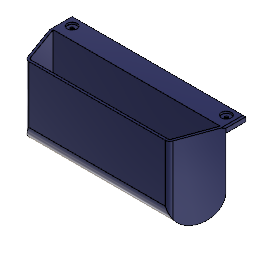
1-Drip tray V3 v4 (Autodesk Fusion 360 design; units mm, degrees)
Autodesk Fusion 360 part; units mm, degrees
mesh "Mesh5" [no effect]
sketch "Sketch3" plane through (0, 0, 10) normal (0, 0, 1) x (-1, 0, 0)
  circle A0 centre (-105, -250) radius 2.75
  circle A1 centre (105, 250) radius 2.75
  circle A2 centre (-105, 250) radius 2.75
  circle A3 centre (105, -250) radius 2.75
  line L0 (-95.6031, -253.4202) -> (-74.3399, -195)
  line L1 (-74.3399, -195) -> (74.3399, -195)
  line L2 (74.3399, -195) -> (95.6031, -253.4202)
  arc A4 (95.6031, -253.4202) -> (115, -250) centre (105, -250) ccw
  line L3 (115, -250) -> (115, 250)
  arc A5 (115, 250) -> (95.6031, 253.4202) centre (105, 250) ccw
  line L4 (95.6031, 253.4202) -> (77.9796, 205)
  line L5 (77.9796, 205) -> (-77.9796, 205)
  line L6 (-77.9796, 205) -> (-95.6031, 253.4202)
  arc A6 (-95.6031, 253.4202) -> (-98.3856, 257.5) centre (-105, 250) ccw
  line L7 (-98.3856, 257.5) -> (-111.6144, 257.5)
  arc A7 (-111.6144, 257.5) -> (-115, 250) centre (-105, 250) ccw
  line L8 (-115, 250) -> (-115, -250)
  arc A8 (-115, -250) -> (-111.6144, -257.5) centre (-105, -250) ccw
  line L9 (-111.6144, -257.5) -> (-98.3856, -257.5)
  arc A9 (-98.3856, -257.5) -> (-95.6031, -253.4202) centre (-105, -250) ccw
  line L10 (105, -250) -> (-105, -250) construction
  line L11 (89, -260) -> (-89, -260)
  line L12 (-89, -239.5) -> (89, -239.5)
  line L13 (89, -260) -> (89, -239.5)
  line L14 (-89, -260) -> (-89, -239.5)
  circle A10 centre (79, -250) radius 5
  line L15 (89, -239.5) -> (74.5263, -199.7338)
  line L16 (-89, -239.5) -> (-74.5256, -199.7319)
  line L17 (69.8278, -196.4439) -> (-69.8278, -196.4439)
  circle A11 centre (79, -250) radius 1.75
  arc A12 (74.5263, -199.7338) -> (69.8278, -196.4439) centre (69.8278, -201.4439) ccw
  line L18 (0, -270) -> (0, -284.4677)
  circle A13 centre (-79, -250) radius 5
  circle A14 centre (-79, -250) radius 1.75
  arc A15 (-69.8278, -196.4439) -> (-74.5256, -199.7319) centre (-69.8278, -201.4439) ccw
  line L19 (85.5724, -237.1) -> (72.271, -200.5546)
  arc A16 (72.271, -200.5546) -> (69.8278, -198.8439) centre (69.8278, -201.4439) ccw
  line L20 (69.8278, -198.8439) -> (-69.8278, -198.8439)
  arc A17 (-69.8278, -198.8439) -> (-72.2713, -200.5554) centre (-69.8278, -201.4439) ccw
  line L21 (-85.5724, -237.1) -> (-72.2713, -200.5554)
  line L22 (-85.5724, -237.1) -> (85.5724, -237.1)
  circle A18 centre (79, -250) radius 2.5
  circle A19 centre (-79, -250) radius 2.5
  line L23 (-89, -245.17) -> (89, -245.17)
  line L24 (-89, -254.33) -> (89, -254.33)
  dimension "d33" = 10
  dimension "d35" = 20.5
  dimension "d36" = 16
  dimension "d37" = 16
  dimension "d38" = 10
  dimension "d39" = 10
  dimension "d45" = 1.4439
  dimension "d46" = 1.4439
  dimension "d47" = -2.4
  dimension "d48" = 3.5
  dimension "d50" = 5
  dimension "d67" = 5.67
  dimension "d68" = 9.16
  dimension "d73" = 5
  constraint coincident A0.centre A8.centre
  constraint coincident L10 A10.centre
  constraint parallel L2 L15
  constraint parallel L0 L16
  constraint perpendicular L3 L17
  constraint concentric A10 A11
  constraint tangent L17 A12
  constraint tangent L15 A12
  constraint perpendicular L11 L18
  constraint symmetric A10 L18 A13
  constraint symmetric A11 L18 A14
  constraint symmetric A12 L18 A15
  constraint concentric A11 A18
  constraint symmetric L18 A18 A19
  constraint coincident L14 L23.start
  constraint coincident L13 L23.end
  constraint perpendicular L13 L23
  constraint coincident L14 L24.start
  constraint coincident L13 L24.end
  constraint perpendicular L13 L24
  measures "d33" distance of L10 L11
  measures "d35" distance of L11 L12
  measures "d36" distance of A3.centre L13
  measures "d37" distance of A0.centre L14
  measures "d38" diameter of A10
  measures "d39" distance of L13 A10.centre
  measures "d45" distance of L2 L15
  measures "d46" distance of L1 L17
  measures "d48" diameter of A11
  measures "d50" radius of A12
  measures "d67" distance of L11 L24
  measures "d68" distance of L23 L24
  measures "d73" diameter of A18
extrude "Extrude2" add sketch "Sketch3" against normal blind 80 contours L12 L15 L16 L17 A12 A15 | L19 A16 L20 A17 L21 L22 makes body 1
extrude "Extrude3" add sketch "Sketch3" against normal blind 6 contours L11 L13 L14 A10 A13 L24 | L13 A10 L23 L24 | L14 A13 L23 L24 | L12 L13 L14 A10 A13 L23 | A10 L23 L24 | A10 L24 | A13 L24 | A13 L23 L24 | A10 L23 | A10 A13 L23 L24 | A13 L23 | A18 | A19 bodies 1
extrude "Extrude4" cut sketch "Sketch3" against normal blind 2 contours A10 L23 L24 | A10 L24 | A13 L24 | A13 L23 L24 | A10 L23 | A13 L23 | A18 | A19 bodies 1
extrude "Extrude6" add sketch "Sketch3" against normal blind 80 separate body contours L19 A16 L20 A17 L21 L22 makes body 2
sketch "Sketch4" plane through (0, 0, 0) normal (1, 0, 0) x (0, 1, 0)
  line L0 (196.4439, 10) -> (196.4439, -70)
  line L1 (196.4439, 10) -> (196.4439, -70)
  line L2 (260, 10) -> (239.5, 10)
  line L3 (239.5, 10) -> (239.5, -70)
  line L4 (239.5, -70) -> (196.4439, -70)
  circle A0 centre (217.9719, -48.4719) radius 21.5281
  line L5 (196.4439, 10) -> (239.5, 10)
  line L6 (239.5, 4) -> (260, 4)
  line L7 (260, 4) -> (260, 10)
  line L8 (260, 10) -> (239.5, 10)
  line L9 (198.8439, 10) -> (198.8439, -70)
  line L10 (237.1, 10) -> (237.1, -70)
  circle A1 centre (217.9719, -48.4719) radius 19.1281
  line L11 (239.5, -48.4719) -> (196, -48.4719)
  point P0 (196.4439, 10)
  point P1 (196.4439, -70)
  point P2 (239.5, 10)
  point P3 (239.5, -70)
  point P4 (239.5, 4)
  point P5 (260, 4)
  point P6 (199.7319, 10)
  point P7 (199.7319, -70)
  point P8 (237.1, 10)
  point P9 (198.8439, 10)
  dimension "d62" = -2.4
  constraint coincident P0 L0.start
  constraint coincident P1 L0.end
  constraint coincident P2 L2.end
  constraint coincident P3 L3.end
  constraint tangent L1 A0
  constraint tangent L4 A0
  constraint tangent L3 A0
  constraint coincident P4 L6.start
  constraint coincident P5 L6.end
  constraint coincident L2.start L7.end
  constraint coincident A0 L11.start
  constraint perpendicular L0 L11
extrude "Extrude5" cut sketch "Sketch4" along normal mid plane 240 contours L0 L1 L4 A0 L9 | L4 A0 L9 | L4 A0 L10 | L3 L4 A0 L10 bodies 1
extrude "Extrude7" cut sketch "Sketch4" along normal mid plane 180 contours L0 L1 L4 A0 L9 | A0 L9 L11 | A0 L9 L10 A1 | L4 A0 L9 | L4 A0 L10 | A0 L10 L11 | L3 L4 A0 L10 picked at (197.2948, -49.3251) picked at (217.9719, -68.3643) picked at (238.6491, -49.3251) bodies 2
combine "Combine1" operation cut target body 1 tool bodies 2
chamfer "Chamfer1" distance 1.4 angle 45 3 edges at (89, 249.75, 10) (0, 260, 10) (-89, 249.75, 10) on bodies 1
extrude "Extrude8" add sketch "Sketch3" against normal blind 1 from surface at -6 separate body contours L13 A10 L23 L24 | L14 A13 L23 L24 | A10 L23 L24 | A13 L23 L24 | A10 A13 L23 L24 makes body 3
chamfer "Chamfer2" distance 1 angle 45 4 edges at (0, 254.33, 3) (89, 249.75, 3) (0, 245.17, 3) (-89, 249.75, 3) on bodies 3
combine "Combine2" operation add target body 3 tool bodies 1
extrude "Extrude9" cut 1 faces at (76.8222, 250.5418, 4) along direction (0, 0, 1) blind 2.8 on bodies 3 bodies 3
extrude "Extrude10" cut 1 faces at (-81.1778, 250.5418, 4) along direction (0, 0, 1) blind 2.8 on bodies 3 bodies 3
equation "d46 = d45"
equation "d67 = 5.42 mm + 0.25 mm"
